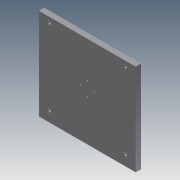
# Autodesk Inventor part: tb2
Saved by Autodesk Inventor 2011 (Build 150239000, 239)
## iProperties
Created: 2011-09-17
Part Number: tb2
Document SubType Name: Modeling
Designer: Matthew
Density: 1 g/cm^3
Author: Matthew
Autodesk Inventor part; units mm, degrees
ref_plane "YZ Plane" through (0, 0, 0) normal (1, 0, 0) x (0, 1, 0)
ref_plane "XZ Plane" through (0, 0, 0) normal (0, 1, 0) x (-1, 0, 0)
ref_plane "XY Plane" through (0, 0, 0) normal (0, 0, 1) x (1, 0, 0)
sketch "Sketch1" plane through (0, 0, 0) normal (0, 0, 1) x (1, 0, 0)
  line L0 (-25.4072, 25.3665) -> (76.1928, 25.3665)
  line L1 (76.1928, 25.3665) -> (76.1928, -76.2335)
  line L2 (76.1928, -76.2335) -> (-25.4072, -76.2335)
  line L3 (-25.4072, -76.2335) -> (-25.4072, 25.3665)
  point P0 (0, 0)
  dimension "d0" = 101.6
  dimension "d1" = 101.6
  constraints: 8 end point, 2 parallel, 1 horizontal, 1 perpendicular
  measures "d0" distance of L1.end L2.end
  measures "d1" distance of L0.end L1.end
extrude "Extrusion1" add sketch "Sketch1" along normal blind 0.7366
sketch "Sketch2" plane through (0, 0, 0.7366) normal (0, 0, 1) x (1, 0, 0)
  line L0 (-25.4072, 25.3665) -> (76.1928, -76.2335)
  line L1 (76.1928, 25.3665) -> (-25.4072, -76.2335)
  circle A0 centre (25.3928, -25.4335) radius 27.432
  point P0 (0, 0)
  dimension "d4" = 54.864
  constraints: 4 end point, 1 centre point, 1 midpoint, 1 perpendicular
  measures "d4" diameter of A0
extrude "Extrusion2" cut sketch "Sketch2" against normal blind 0.7366
sketch "Sketch3" plane through (0, 0, 0.7366) normal (0, 0, 1) x (1, 0, 0)
  line L0 (-25.4072, -76.2335) -> (-25.4072, 25.3665) projected
  line L1 (-25.4072, 25.3665) -> (-25.4072, -25.4335)
  line L2 (-25.4072, -25.4335) -> (-25.4072, 19.4102)
  line L3 (-25.4072, 25.3665) -> (76.1928, -76.2335)
  line L4 (76.1928, 25.3665) -> (-25.4072, -76.2335)
  circle A0 centre (-19.4509, 19.4102) radius 1.9812
  point P0 (0, 0)
  dimension "d7" = 44.8437
  dimension "d8" = 3.9624
  constraints: 8 end point, 2 point on line, 1 centre point, 1 midpoint, 1 perpendicular
  measures "d7" distance of L1.end L2.end
  measures "d8" diameter of A0
extrude "Extrusion3" cut sketch "Sketch3" against normal blind 0.7366 contours A0 L3 | L3 A0
sketch "Sketch4" plane through (0, 0, 0.7366) normal (0, 0, 1) x (1, 0, 0)
  line L0 (-25.4072, -76.2335) -> (76.1928, 25.3665)
  line L1 (-25.4072, 25.3665) -> (76.1928, -76.2335)
  circle A0 centre (70.2365, 19.4102) radius 1.9819
  circle A1 centre (70.2365, -70.2772) radius 1.983
  circle A2 centre (-19.4509, -70.2772) radius 1.9812
  point P0 (0, 0)
  constraints: 4 end point, 3 centre point, 3 point on line, 1 perpendicular
extrude "Extrusion4" cut sketch "Sketch4" against normal blind 0.7366
sketch "Sketch5" plane through (0, 0, 0.7366) normal (0, 0, 1) x (1, 0, 0)
  circle A0 centre (25.3928, -25.4335) radius 27.432 projected
  circle A1 centre (25.3928, -25.4335) radius 29.972
  circle A2 centre (25.3928, -25.4335) radius 32.512
  point P0 (0, 0)
  dimension "d13" = 59.944
  dimension "d14" = 65.024
  constraints: 2 centre point, 2 coincident
  measures "d13" diameter of A1
  measures "d14" diameter of A2
extrude "Extrusion5" add sketch "Sketch5" along normal blind 6.6548 contours A2
fillet "Fillet1" radius 3.175 4 edges at (-25.4072, 25.3665, 0.3683) (76.1928, 25.3665, 0.3683) (76.1928, -76.2335, 0.3683) (-25.4072, -76.2335, 0.3683)
sketch "Sketch6" plane through (0, 0, 0) normal (0, 0, -1) x (-1, 0, 0)
  circle A0 centre (-70.2365, 19.4102) radius 1.9819 projected
  circle A1 centre (19.4509, -70.2772) radius 1.9812 projected
  circle A2 centre (-70.2365, -70.2772) radius 1.983 projected
  circle A3 centre (19.4509, 19.4102) radius 1.9812 projected
  line L0 (-76.1928, 25.3665) -> (25.4072, 25.3665)
  line L1 (25.4072, 25.3665) -> (25.4072, -76.2335)
  line L2 (25.4072, -76.2335) -> (-76.1928, -76.2335)
  line L3 (-76.1928, -76.2335) -> (-76.1928, 25.3665)
  point P0 (0, 0)
  constraints: 8 end point, 2 parallel, 1 horizontal, 1 perpendicular
extrude "Extrusion6" add sketch "Sketch6" against normal blind 6.35
sketch "Sketch7" plane through (0, 0, 6.35) normal (0, 0, 1) x (1, 0, 0)
  line L0 (-14.3145, 13.5707) -> (65.0173, 13.5707)
  line L1 (65.0173, 13.5707) -> (65.0173, -65.16)
  line L2 (65.0173, -65.16) -> (-14.3145, -65.16)
  line L3 (-14.3145, -65.16) -> (-14.3145, 13.5707)
  point P0 (0, 0)
  constraints: 8 end point, 2 parallel, 1 horizontal, 1 perpendicular
extrude "Extrusion7" cut sketch "Sketch7" along normal blind 6.35
sketch "Sketch8" plane through (0, 0, 6.35) normal (0, 0, 1) x (1, 0, 0)
  circle A0 centre (70.2365, -70.2772) radius 1.983 projected
  circle A1 centre (-19.4509, 19.4102) radius 1.9812 projected
  line L0 (-19.4509, 19.4102) -> (70.2365, 19.4102)
  line L1 (70.2365, 19.4102) -> (70.2365, -70.2772)
  line L2 (70.2365, -70.2772) -> (-19.4509, -70.2772)
  line L3 (-19.4509, -70.2772) -> (-19.4509, 19.4102)
  line L4 (63.8865, 13.0602) -> (-13.1009, 13.0602)
  line L5 (-13.1009, 13.0602) -> (-13.1009, -63.9272)
  line L6 (-13.1009, -63.9272) -> (63.8865, -63.9272)
  line L7 (63.8865, -63.9272) -> (63.8865, 13.0602)
  line L8 (-13.1009, -25.4335) -> (-13.1009, -19.0835)
  line L9 (-13.1009, -19.0835) -> (63.8865, -19.0835)
  line L10 (63.8865, -19.0835) -> (63.8865, -31.7835)
  line L11 (63.8865, -31.7835) -> (-13.1009, -31.7835)
  point P0 (0, 0)
  dimension "d22" = 6.35
  dimension "d23" = 6.35
  dimension "d24" = 12.7
  constraints: 24 end point, 4 parallel, 4 perpendicular, 4 point on line, 1 horizontal, 1 midpoint, 3 other
  measures "d22" distance between parallel lines of L0 L4
  measures "d23" distance of L8.start L8.end
  measures "d24" distance of L9.end L10.end
extrude "Extrusion8" cut sketch "Sketch8" against normal blind 25.4 contours L7 L9 L5 L4 | L7 L6 L5 L11
sketch "Sketch9" plane through (0, 0, 6.35) normal (0, 0, 1) x (1, 0, 0)
  line L0 (63.8865, -63.9272) -> (-13.1009, -63.9272) projected
  line L1 (-13.1009, 13.0602) -> (63.8865, 13.0602) projected
  line L2 (-25.4072, 25.3665) -> (76.1928, 25.3665) projected
  line L3 (76.1928, -76.2335) -> (-25.4072, -76.2335) projected
  line L4 (-13.1009, 13.0602) -> (-13.1009, 25.3665)
  line L5 (63.8865, 13.0602) -> (63.8865, 25.3665)
  line L6 (63.8865, -63.9272) -> (63.8865, -76.2335)
  line L7 (-13.1009, -63.9272) -> (-13.1009, -76.2335)
  point P0 (0, 0)
  constraints: 8 end point, 4 point on line, 2 parallel, 2 perpendicular
extrude "Extrusion9" cut sketch "Sketch9" against normal blind 25.4
sketch "Sketch10" plane through (0, 0, 6.35) normal (0, 0, 1) x (1, 0, 0)
  line L0 (-13.1009, 25.3665) -> (63.8865, 25.3665)
  line L1 (63.8865, 25.3665) -> (63.8865, -76.2335)
  line L2 (63.8865, -76.2335) -> (-13.1009, -76.2335)
  line L3 (-13.1009, -76.2335) -> (-13.1009, 25.3665)
  point P0 (0, 0)
  constraints: 8 end point, 2 parallel, 1 horizontal, 1 perpendicular
extrude "Extrusion10" add sketch "Sketch10" against normal blind 6.35
sketch "Sketch11" plane through (76.1928, -76.2335, 0) normal (1, 0, 0) x (0, 0, -1)
  line L0 (0, 101.6) -> (0, 0) projected
  line L1 (0, 101.6) -> (-6.35, 101.6) projected
  line L2 (-6.35, 101.6) -> (-6.35, 0) projected
  line L3 (0, 0) -> (-6.35, 0) projected
  point P0 (0, 76.2335)
extrude "Extrusion11" add sketch "Sketch11" along normal blind 6.35
sketch "Sketch12" plane through (-25.4072, -76.2335, 0) normal (-1, 0, 0) x (0, 0, 1)
  line L0 (0, 0) -> (0, 101.6) projected
  line L1 (0, 0) -> (6.35, 0) projected
  line L2 (6.35, 0) -> (6.35, 101.6) projected
  line L3 (0, 101.6) -> (6.35, 101.6) projected
  point P0 (0, 76.2335)
extrude "Extrusion12" add sketch "Sketch12" along normal blind 6.35
sketch "Sketch13" plane through (82.5428, -76.2335, 0) normal (0, -1, 0) x (1, 0, 0)
  line L0 (0, 6.35) -> (-114.3, 6.35) projected
  line L1 (-114.3, 6.35) -> (-114.3, 0) projected
  line L2 (0, 0) -> (-114.3, 0) projected
  line L3 (0, 0) -> (0, 6.35) projected
  point P0 (-82.5428, 0)
extrude "Extrusion13" add sketch "Sketch13" along normal blind 6.35
sketch "Sketch14" plane through (0, 0, 0) normal (0, 0, -1) x (-1, 0, 0)
  circle A0 centre (19.4509, 19.4102) radius 1.9812 projected
  circle A1 centre (19.4509, -70.2772) radius 1.9812 projected
  line L0 (-82.5428, -82.5835) -> (31.7572, -82.5835) projected
  line L1 (19.4509, -70.2772) -> (19.4509, 19.4102)
  line L2 (19.4509, -25.4335) -> (-25.3928, -25.4335)
  circle A2 centre (-25.3928, -25.4335) radius 8
  circle A3 centre (-25.3928, -33.4335) radius 1
  circle A4 centre (-33.3928, -25.4335) radius 1
  circle A5 centre (-17.3928, -25.4335) radius 1
  circle A6 centre (-25.3928, -17.4335) radius 1
  point P0 (0, 0)
  dimension "d37" = 16
  dimension "d38" = 2
  dimension "d39" = 2
  dimension "d40" = 2
  dimension "d41" = 2
  constraints: 5 centre point, 4 end point, 4 point on circle, 2 perpendicular, 1 coincident, 1 midpoint, 1 point on line
  measures "d37" diameter of A2
  measures "d38" diameter of A3
  measures "d39" diameter of A4
  measures "d40" diameter of A5
  measures "d41" diameter of A6
extrude "Extrusion14" cut sketch "Sketch14" against normal blind 25.4 contours A5 A2 L2 | L2 A2 A5 | A2 A5 L2 | L2 A5 A2 | A6 A2 | A2 A6 | A3 A2 | A2 A3 | A4 A2 | A2 A4
body "Solid1"
